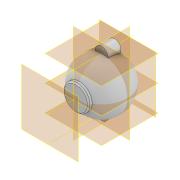
# Autodesk Inventor part: Hips
Saved by Autodesk Inventor 2021 (Build 250183000, 183)
## iProperties
Created: 2020-12-19
Part Number: Hips
Material: 一般
Document SubType Name: Modeling
Designer: Tazaki
Density: 2.29325 g/cm^3
Appearance: 既定
Mass: 10000 g
Surface Area: 1381.04 cm^2
Volume: 4360.62 cm^3
Author: Tazaki
Autodesk Inventor part; units mm, degrees
sketch "スケッチ1" plane through (0, 0, 0) normal (0, 0, 1) x (1, 0, 0)
  arc A0 (0, 100) -> (0, -100) centre (0, 0) ccw
  line L0 (0, 100) -> (0, -100)
  dimension "d0" = 200
  constraints: 2 end point, 2 point on circle, 1 centre point, 1 coincident, 1 vertical
  measures "d0" diameter of A0
revolve "回転1" add sketch "スケッチ1" angle 360 about axis through (0, 100, 0) along (0, -1, 0)
ref_plane "作業平面1" through (0, 0, 200) normal (0, 0, 1) x (1, 0, 0)
ref_plane "作業平面2" through (0, 100, 0) normal (0, 1, 0) x (-1, 0, 0)
ref_plane "作業平面3" through (0, -100, 0) normal (0, 1, 0) x (-1, 0, 0)
ref_plane "作業平面4" through (0, 0, -100) normal (0, 0, 1) x (1, 0, 0)
sketch "スケッチ2" plane through (0, 0, 0) normal (0, 0, 1) x (1, 0, 0)
  circle A0 centre (0, 0) radius 50
  dimension "d6" = 100
  constraints: 1 centre point, 1 coincident
  measures "d6" diameter of A0
extrude "押し出し1" add sketch "スケッチ2" along normal blind 100
chamfer "面取り1" distance 5 angle 45 1 edges at (-50, 0, 100)
sketch "スケッチ3" plane through (0, 0, 0) normal (0, 0, 1) x (1, 0, 0)
  circle A0 centre (0, 100) radius 25
  point P0 (0, 0)
  dimension "d12" = 50
  dimension "d13" = 100
  constraints: 1 centre point, 1 vertical alignment
  measures "d12" diameter of A0
  measures "d13" distance of point (0, 0) A0.centre
extrude "押し出し2" add sketch "スケッチ3" against normal blind 50
mirror "ミラー1" about plane through (0, 0, 0) normal (0, 1, 0) of "押し出し2"
